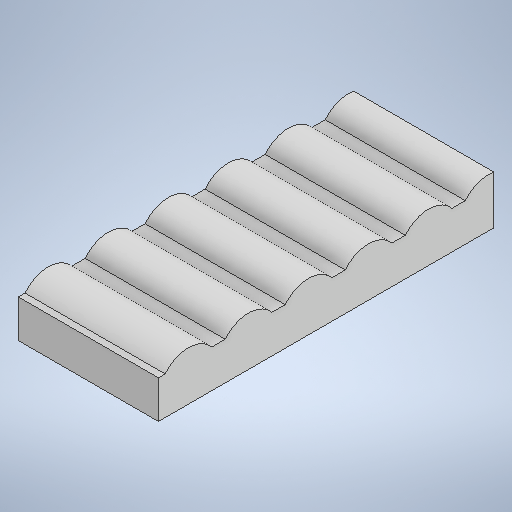
# Autodesk Inventor part: Pad
Saved by Autodesk Inventor 2027 (Build 310192060, 192F)
## iProperties
Created: 2026-07-01
Part Number: Pad
Material: Generic
Document SubType Name: Modeling
Designer: 13129
Density: 1 g/cm^3
Appearance: Default
Author: 13129
Autodesk Inventor part; units mm, degrees
ref_plane "YZ Plane" through (0, 0, 0) normal (1, 0, 0) x (0, 1, 0)
ref_plane "XZ Plane" through (0, 0, 0) normal (0, 1, 0) x (-1, 0, 0)
ref_plane "XY Plane" through (0, 0, 0) normal (0, 0, 1) x (1, 0, 0)
sketch "Sketch1" plane through (0, 0, 0) normal (0, 1, 0) x (-1, 0, 0)
  line L0 (0, 0) -> (0, -70.92)
  line L1 (0, -70.92) -> (29.645, -70.92)
  line L2 (29.645, -70.92) -> (29.645, 0)
  line L3 (29.645, 0) -> (0, 0)
  dimension "d0" = 70.92
  dimension "d1" = 29.645
  constraints: 8 end point, 2 perpendicular, 1 horizontal, 1 horizontal alignment, 1 vertical
  measures "d0" distance of L0.start L0.end
  measures "d1" distance of L0.end L1.end
extrude "Extrusion1" add sketch "Sketch1" along normal blind 8
sketch "Sketch2" plane through (0, 0, 0) normal (1, 0, 0) x (0, 0, -1)
  line L0 (0, 0) -> (70.92, 0) construction
  line L1 (0, 8) -> (70.92, 8) construction
  line L2 (0, 0) -> (0, 8) construction
  circle A0 centre (6.35, 4) radius 6.35
  circle A1 centre (19.05, 4) radius 6.35
  circle A2 centre (31.75, 4) radius 6.35
  circle A3 centre (44.45, 4) radius 6.35
  circle A4 centre (57.15, 4) radius 6.35
  circle A5 centre (69.85, 4) radius 6.35
  line L3 (70.92, 0) -> (0, 0) construction
  line L4 (70.92, 0) -> (70.92, -2.2592)
  line L5 (70.92, 0) -> (70.92, 8) construction
  line L6 (70.92, 8) -> (70.92, 10.2592)
  line L7 (70.92, 8) -> (0, 8)
  point P0 (0, 4)
  point P1 (0, 4)
  point P2 (64.9182, 8)
  point P3 (52.2182, 8)
  point P4 (62.0818, 8)
  point P5 (39.5182, 8)
  point P6 (49.3818, 8)
  point P7 (26.8182, 8)
  point P8 (36.6818, 8)
  point P9 (14.1182, 8)
  point P10 (23.9818, 8)
  point P11 (1.4182, 8)
  point P12 (11.2818, 8)
  dimension "d4" = 6.35
  dimension "d7" = 12.7
  constraints: 6 centre point, 6 end point, 2 midpoint, 2 point on circle, 2 vertical, 1 collinear, 1 horizontal, 1 horizontal alignment, 1 tangent, 10 other
  measures "d4" distance of point (0, 4) A0.centre
  measures "d7" distance of A0.centre A1.centre
extrude "Extrusion2" add sketch "Sketch2" against normal up to surface (29.645 mm away) contours L7 A0 | A1 L7 | A2 L7 | A3 L7 | A4 L7 | A5 L6 L7 picked at (6.8167, 8.7312) picked at (18.1395, 8.5775) picked at (33.0595, 8.3297) picked at (43.205, 8.9072) picked at (55.905, 8.9072) picked at (67.2357, 8.3157)
body "Solid1"
